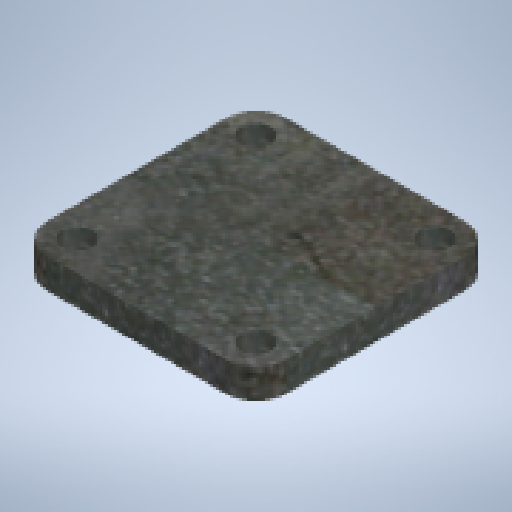
# Autodesk Inventor part: part6
Saved by Autodesk Inventor 2025.2 (Build 292293000, 293)
## iProperties
Created: 2024-12-09
Part Number: part6
Material: Stal
Document SubType Name: Modeling
Designer: Marek
Density: 7.85 g/cm^3
Appearance: Płyta
Author: Marek
Autodesk Inventor part; units mm, degrees
ref_plane "YZ Plane" through (0, 0, 0) normal (1, 0, 0) x (0, 1, 0)
ref_plane "XZ Plane" through (0, 0, 0) normal (0, 1, 0) x (-1, 0, 0)
ref_plane "XY Plane" through (0, 0, 0) normal (0, 0, 1) x (1, 0, 0)
sketch "Szkic1" plane through (0, 0, 0) normal (0, 1, 0) x (-1, 0, 0)
  line L0 (-15, 20) -> (15, 20)
  line L1 (20, 15) -> (20, -15)
  line L2 (15, -20) -> (-15, -20)
  line L3 (-20, -15) -> (-20, 15)
  line L4 (-20, 20) -> (20, -20) construction
  line L5 (20, 20) -> (-20, -20) construction
  arc A0 (-15, 20) -> (-20, 15) centre (-15, 15) ccw
  arc A1 (20, 15) -> (15, 20) centre (15, 15) ccw
  arc A2 (15, -20) -> (20, -15) centre (15, -15) ccw
  arc A3 (-20, -15) -> (-15, -20) centre (-15, -15) ccw
  circle A4 centre (15, -15) radius 2.5
  circle A5 centre (-15, -15) radius 2.5
  circle A6 centre (-15, 15) radius 2.5
  circle A7 centre (15, 15) radius 2.5
  point P0 (0, 0)
  dimension "d0" = 40
  dimension "d1" = 40
  dimension "d2" = 5
  dimension "d3" = 5
  constraints: 12 end point, 8 centre point, 8 point on circle, 8 point on line, 8 tangent, 6 equal radius, 4 coincident, 2 midpoint, 2 parallel, 1 horizontal, 1 perpendicular
  measures "d0" distance of L4.end L5.end
  measures "d1" distance of L5.start L4.end
  measures "d2" radius of A0
  measures "d3" diameter of A4
extrude "Wyciągnięcie proste1" add sketch "Szkic1" along normal blind 5
